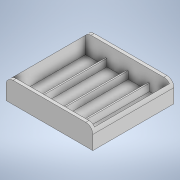
# Autodesk Inventor part: RoughBatteryPack
Saved by Autodesk Inventor 2020 (Build 240168000, 168)
## iProperties
Created: 2023-02-04
Part Number: RoughBatteryPack
Material: Generic
Document SubType Name: Modeling
Designer: legoo
Density: 1 g/cm^3
Appearance: Default
Author: legoo
Autodesk Inventor part; units mm, degrees
ref_plane "YZ Plane" through (0, 0, 0) normal (1, 0, 0) x (0, 1, 0)
ref_plane "XZ Plane" through (0, 0, 0) normal (0, 1, 0) x (-1, 0, 0)
ref_plane "XY Plane" through (0, 0, 0) normal (0, 0, 1) x (1, 0, 0)
sketch "Sketch1" plane through (0, 0, 0) normal (0, 1, 0) x (-1, 0, 0)
  line L0 (0, 0) -> (62, 0)
  line L1 (62, 0) -> (62, -58)
  line L2 (62, -58) -> (0, -58)
  line L3 (0, -58) -> (0, 0)
  dimension "d0" = 62
  dimension "d1" = 58
  constraints: 8 end point, 2 parallel, 1 horizontal, 1 perpendicular
  measures "d0" distance of L1.end L2.end
  measures "d1" distance of L0.end L1.end
extrude "Extrusion1" add sketch "Sketch1" along normal blind 15
sketch "Sketch2" plane through (0, 0, -58) normal (0, 0, -1) x (-1, 0, 0)
  line L0 (62, 0) -> (0, 0) projected
  line L1 (0, 0) -> (62, 0)
  line L2 (62, 0) -> (62, 10)
  line L3 (57, 15) -> (5, 15)
  line L4 (0, 10) -> (0, 0)
  arc A0 (5, 15) -> (0, 10) centre (5, 10) ccw
  arc A1 (62, 10) -> (57, 15) centre (57, 10) ccw
  line L5 (0, 10) -> (-2.4331, 10)
  line L6 (-2.4331, 10) -> (-2.4331, 19.594)
  line L7 (-2.4331, 19.594) -> (72.365, 19.594)
  line L8 (72.365, 19.594) -> (72.365, 10)
  line L9 (72.365, 10) -> (62, 10)
  point P0 (62, 15)
  dimension "d4" = 5
  constraints: 18 end point, 5 perpendicular, 4 point on circle, 4 tangent, 3 point on line, 2 centre point, 2 horizontal, 2 parallel, 1 equal radius
  measures "d4" radius of A0
extrude "Extrusion2" cut sketch "Sketch2" against normal up to surface (58 mm away) contours A1 L3 A0 L5 L6 L7 L8 L9
sketch "Sketch3" plane through (0, 15, 0) normal (0, 1, 0) x (1, 0, 0)
  line L0 (-1, 2.25) -> (-61, 2.25)
  line L1 (-61, 2.25) -> (-61, 55.75)
  line L2 (-61, 55.75) -> (-1, 55.75)
  line L3 (-1, 55.75) -> (-1, 2.25)
  line L4 (-57, 0) -> (-5, 0) projected
  line L5 (-5, 58) -> (-57, 58) projected
  line L6 (-62, 0) -> (-62, 58) projected
  line L7 (0, 58) -> (0, 0) projected
  dimension "d7" = 2.25
  dimension "d8" = 2.25
  dimension "d9" = 1
  dimension "d10" = 1
  constraints: 8 end point, 2 parallel, 1 horizontal, 1 perpendicular
  measures "d7" distance between parallel lines of L0 L4
  measures "d8" distance between parallel lines of L5 L2
  measures "d9" distance between parallel lines of L6 L1
  measures "d10" distance between parallel lines of L7 L3
extrude "Extrusion3" cut sketch "Sketch3" against normal blind 14
sketch "Sketch4" plane through (0, 1, 0) normal (0, 1, 0) x (1, 0, 0)
  line L0 (-5, 2.25) -> (-57, 2.25) projected
  line L1 (-57, 55.75) -> (-5, 55.75) projected
  line L2 (-15.25, 2.25) -> (-16.25, 2.25)
  line L3 (-16.25, 2.25) -> (-16.25, 55.75)
  line L4 (-16.25, 55.75) -> (-15.25, 55.75)
  line L5 (-15.25, 55.75) -> (-15.25, 2.25)
  line L6 (-30.5, 2.25) -> (-31.5, 2.25)
  line L7 (-31.5, 2.25) -> (-31.5, 55.75)
  line L8 (-31.5, 55.75) -> (-30.5, 55.75)
  line L9 (-30.5, 55.75) -> (-30.5, 2.25)
  line L10 (-45.75, 2.25) -> (-46.75, 2.25)
  line L11 (-46.75, 2.25) -> (-46.75, 55.75)
  line L12 (-46.75, 55.75) -> (-45.75, 55.75)
  line L13 (-45.75, 55.75) -> (-45.75, 2.25)
  line L14 (-61, 2.25) -> (-61, 55.75) projected
  line L15 (-1, 55.75) -> (-1, 2.25) projected
  point P0 (0, 0)
  dimension "d13" = 1
  dimension "d14" = 1
  dimension "d15" = 1
  dimension "d16" = 14.25
  dimension "d17" = 14.25
  dimension "d18" = 14.25
  constraints: 24 end point, 6 parallel, 6 point on line, 3 horizontal, 3 perpendicular
  measures "d13" distance between parallel lines of L3 L5
  measures "d14" distance between parallel lines of L7 L9
  measures "d15" distance between parallel lines of L11 L13
  measures "d16" distance between parallel lines of L14 L11
  measures "d17" distance between parallel lines of L15 L5
  measures "d18" distance between parallel lines of L9 L3
extrude "Extrusion4" add sketch "Sketch4" along normal blind 5.25 contours L0 L3 L1 L5 | L0 L7 L1 L9 | L0 L11 L1 L13
body "Solid1"
